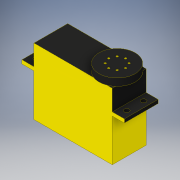
# Autodesk Inventor part: servo
Saved by Autodesk Inventor 2019 (Build 230136000, 136)
## iProperties
Created: 2019-02-02
Part Number: servo
Material: Aluminum
Document SubType Name: Modeling
Designer: suchanek
Density: 2.7 g/cm^3
Appearance: Satin
Author: suchanek
Autodesk Inventor part; units mm, degrees
ref_plane "YZ Plane" through (0, 0, 0) normal (1, 0, 0) x (0, 1, 0)
ref_plane "XZ Plane" through (0, 0, 0) normal (0, 1, 0) x (-1, 0, 0)
ref_plane "XY Plane" through (0, 0, 0) normal (0, 0, 1) x (1, 0, 0)
sketch "Sketch1" plane through (0, 0, 0) normal (0, 1, 0) x (-1, 0, 0)
  line L0 (32.5, 14) -> (19.5, 14)
  line L1 (-32.5, 14) -> (-32.5, -14)
  line L2 (-32.5, -14) -> (19.5, -14)
  line L3 (32.5, -14) -> (32.5, 14)
  line L4 (32.5, 14) -> (-32.5, -14) construction
  line L5 (-32.5, 14) -> (32.5, -14) construction
  line L6 (19.5, 14) -> (-32.5, 14)
  line L7 (19.5, -14) -> (32.5, -14)
  point P0 (0, 0)
  point P1 (32.5, 7.3274)
  point P2 (32.5, -11.3274)
  dimension "d0" = 65
  dimension "d1" = 28
  constraints: 16 end point, 5 parallel, 2 horizontal, 2 midpoint, 2 perpendicular, 2 point on line, 1 vertical alignment
  measures "d0" distance of L0.start L1.start
  measures "d1" distance of L3.start L0.start
extrude "Extrusion1" add sketch "Sketch1" along normal blind 55
sketch "Sketch2" plane through (0, 55, 0) normal (0, 1, 0) x (1, 0, 0)
  circle A0 centre (22.5, 0) radius 15
  line L0 (32.5, -14) -> (32.5, 14) projected
  line L1 (-32.5, -14) -> (32.5, -14) projected
  point P0 (0, 0)
  point P1 (-8.5, -16)
  dimension "d4" = 10
  dimension "d5" = 30
  dimension "d28" = 14
  constraints: 1 centre point, 1 other
  measures "d4" distance from line of L0 A0.centre
  measures "d5" diameter of A0
extrude "Extrusion2" add sketch "Sketch2" along normal blind 6 contours A0 L0 | L0 A0 L1 | L1 A0 picked at (24.6253, 2.0919)
sketch "Sketch3" plane through (22.5, 61, 0) normal (0, 1, 0) x (1, 0, 0)
  circle A0 centre (-7, 0) radius 0.8
  circle A1 centre (0, 0) radius 15 projected
  circle A2 centre (-4.9497, -4.9497) radius 0.8
  circle A3 centre (0, -7) radius 0.8
  circle A4 centre (4.9497, -4.9497) radius 0.8
  circle A5 centre (7, 0) radius 0.8
  circle A6 centre (4.9497, 4.9497) radius 0.8
  circle A7 centre (0, 7) radius 0.8
  circle A8 centre (-4.9497, 4.9497) radius 0.8
  point P0 (-22.5, 0)
  dimension "d12" = 1.6
  dimension "d14" = 7
  dimension "d17" = 360
  constraints: 8 centre point, 1 coincident, 1 horizontal alignment, 17 other
  measures "d12" diameter of A0
  measures "d14" distance of A1.centre A0.centre
extrude "Extrusion3" cut sketch "Sketch3" against normal up to surface (6 mm away) contours A0 | A2 | A3 | A4 | A5 | A6 | A7 | A8
sketch "Sketch4" plane through (0, 55, 0) normal (0, 1, 0) x (1, 0, 0)
  circle A0 centre (-37.5, -7) radius 2
  circle A1 centre (37.5, -7) radius 2
  circle A2 centre (37.5, 7) radius 2
  circle A3 centre (-37.5, 7) radius 2
  line L0 (-32.5, -14) -> (32.5, -14) projected
  line L1 (32.5, -14) -> (32.5, 14) projected
  line L2 (-32.5, 14) -> (-32.5, -14) projected
  line L3 (-32.5, 14) -> (-42.5, 14)
  line L4 (-42.5, 14) -> (-42.5, -14)
  line L5 (-42.5, -14) -> (-32.5, -14)
  line L6 (-32.5, -14) -> (-32.5, 14)
  line L7 (32.5, 14) -> (42.5, 14)
  line L8 (42.5, 14) -> (42.5, -14)
  line L9 (42.5, -14) -> (32.5, -14)
  line L10 (32.5, -14) -> (32.5, 14)
  point P0 (0, 0)
  point P1 (-8.5, -16)
  point P2 (29.5, -14)
  point P3 (32.5, -11)
  point P4 (32.5, 11)
  dimension "d21" = 4
  dimension "d22" = 14
  dimension "d23" = 7
  dimension "d29" = 5
  dimension "d30" = 5
  dimension "d31" = 5
  dimension "d32" = 5
  constraints: 16 end point, 4 centre point, 4 parallel, 3 equal radius, 3 horizontal, 2 horizontal alignment, 2 perpendicular, 2 vertical alignment, 1 point on line, 1 other
  measures "d21" diameter of A3
  measures "d22" distance of A1.centre A2.centre
  measures "d29" distance from line of L1 A1.centre
  measures "d30" distance from line of A0.centre L2
  measures "d31" distance from line of L4 A0.centre
  measures "d32" distance from line of L8 A1.centre
extrude "Extrusion4" add sketch "Sketch4" against normal blind 20
sketch "Sketch5" plane through (0, 55, 0) normal (0, 1, 0) x (1, 0, 0)
  line L0 (42.5, 14) -> (-42.5, 14) projected
  line L1 (-32.5, 14) -> (-32.5, -14) projected
  line L2 (-42.5, 14) -> (-32.5, 14)
  line L3 (-32.5, 14) -> (-32.5, -14)
  line L4 (-32.5, -14) -> (-42.5, -14)
  line L5 (-42.5, -14) -> (-42.5, 14)
  line L6 (32.5, -14) -> (32.5, 14) projected
  line L7 (42.5, 14) -> (42.5, -14) projected
  line L8 (32.5, -14) -> (42.5, -14)
  line L9 (42.5, -14) -> (42.5, 14)
  line L10 (42.5, 14) -> (32.5, 14)
  line L11 (32.5, 14) -> (32.5, -14)
  point P0 (0, 0)
  constraints: 16 end point, 4 parallel, 2 horizontal, 2 perpendicular
extrude "Extrusion5" cut sketch "Sketch5" against normal blind 17
equation "\"d30\" = d29"
equation "\"d31\" = d30"
equation "\"d32\" = d29"
body "Solid1"
